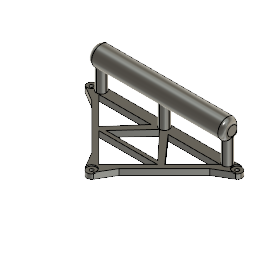
top handle v4 (Autodesk Fusion 360 design; units mm, degrees)
Autodesk Fusion 360 part; units mm, degrees
note: some values were not read from the file. Chosen so that the rebuilt part matches the saved one: which face or edge a step refers to; which pieces of a blend or face edit are solid. Set by a fixed rule: which sketch regions a step uses.
sketch "Sketch1" plane through (0, 0, 0) normal (0, 0, 1) x (1, 0, 0)
  circle A0 centre (0, 0) radius 1.5
  line L0 (0, 0) -> (120, 0)
  circle A1 centre (120, 0) radius 1.5
  circle A2 centre (120, 0) radius 4
  circle A3 centre (0, 0) radius 4
  line L1 (0, 4) -> (0, -4)
  line L2 (120, 4) -> (120, -4)
  line L3 (0, 4) -> (0, -4)
  line L4 (0, -4) -> (9, -4)
  line L5 (9, 4) -> (0, 4)
  line L6 (120, 4) -> (120, -4)
  line L7 (120, -4) -> (111, -4)
  line L8 (111, 4) -> (120, 4)
  line L9 (60, 0) -> (60, -60)
  line L10 (60, -60) -> (120, 0)
  line L11 (0, 0) -> (60, -60)
  line L12 (60, -60) -> (60, -54)
  line L13 (114, 0) -> (60, -54)
  line L14 (6, 0) -> (60, -54)
  line L15 (9, 4) -> (111, 4)
  line L16 (9, -4) -> (111, -4)
  line L17 (60, 0) -> (60, 4)
  circle A4 centre (60, -60) radius 1.5
  circle A5 centre (60, -60) radius 4
  line L18 (0, 0) -> (11.3137, -11.3137)
  line L19 (11.3137, -11.3137) -> (-2.0315, -3.4457)
  line L20 (120, 0) -> (108.6863, -11.3137)
  line L21 (108.6863, -11.3137) -> (122.0315, -3.4457)
  line L22 (60, -60) -> (71.3137, -48.6863)
  line L23 (71.3137, -48.6863) -> (63.4457, -62.0315)
  line L24 (60, -60) -> (48.6863, -48.6863)
  line L25 (48.6863, -48.6863) -> (56.5543, -62.0315)
  line L26 (0, 0) -> (60, -60)
  line L27 (30, -30) -> (60, 4)
  line L28 (30, -30) -> (33.0052, -33.0052)
  line L29 (33.0052, -33.0052) -> (60, -4)
  line L30 (60, -60) -> (120, 0)
  line L31 (90, -30) -> (60, 4)
  line L32 (90, -30) -> (86.9948, -33.0052)
  line L33 (60, -4) -> (86.9948, -33.0052)
  line L34 (35.8975, -29.8975) -> (84.1025, -29.8975)
  line L35 (87.1875, -26.8125) -> (32.8125, -26.8125)
  line L36 (0, 4) -> (12, 4)
  line L37 (12, 4) -> (12, -4)
  line L38 (12, -4) -> (0, -4)
  line L39 (0, -4) -> (0, 4)
  line L40 (12, 4) -> (4, 4)
  line L41 (4, 4) -> (4, -4)
  line L42 (4, -4) -> (12, -4)
  line L43 (12, -4) -> (12, 4)
  line L44 (120, 4) -> (108, 4)
  line L45 (108, 4) -> (108, -4)
  line L46 (108, -4) -> (120, -4)
  line L47 (120, -4) -> (120, 4)
  line L48 (108, 4) -> (116, 4)
  line L49 (116, 4) -> (116, -4)
  line L50 (116, -4) -> (108, -4)
  line L51 (108, -4) -> (108, 4)
  line L52 (64, -4) -> (56, -4)
  line L53 (56, -4) -> (56, 4)
  line L54 (56, 4) -> (64, 4)
  line L55 (64, 4) -> (64, -4)
  line L56 (64, -4) -> (56, 4) construction
  line L57 (56, -4) -> (64, 4) construction
  point P0 (60, 0)
  dimension "d1" = 3
  dimension "d2" = 120
  dimension "d3" = 3
  dimension "d4" = 8
  dimension "d5" = 8
  dimension "d6" = 9
  dimension "d8" = 9
  dimension "d10" = 60
  dimension "d11" = 6
  dimension "d13" = 3
  dimension "d14" = 8
  dimension "d15" = 16
  dimension "d16" = 16
  dimension "d17" = 16
  dimension "d18" = 16
  dimension "d19" = 4.25
  dimension "d20" = 4.25
  dimension "d25" = 12
  dimension "d26" = 8
  dimension "d27" = 8
  dimension "d28" = 12
  dimension "d29" = 8
  dimension "d39" = 8
  constraint coincident A0.centre L0.start
  constraint horizontal L0
  constraint coincident L0.end A1.centre
  constraint concentric A0 A3
  constraint coincident A3 L1.start
  constraint coincident A3 L1.end
  constraint perpendicular L0 L1
  constraint coincident A2 L2.start
  constraint coincident A2 L2.end
  constraint perpendicular L0 L2
  constraint perpendicular L3 L4
  constraint parallel L4 L5
  constraint parallel L1 L3
  constraint perpendicular L6 L7
  constraint parallel L7 L8
  constraint midpoint L0 P0
  constraint perpendicular L0 L9
  constraint parallel L9 L12
  constraint perpendicular L13 L14
  constraint midpoint L15 L17.end
  constraint perpendicular L15 L17
  constraint coincident L9.end L10.start
  constraint parallel L11 L18
  constraint coincident A3 L19.end
  constraint tangent A3 L19
  constraint parallel L10 L20
  constraint coincident A2 L21.end
  constraint tangent A2 L21
  constraint perpendicular L11 L22
  constraint coincident A5 L23.end
  constraint tangent A5 L23
  constraint perpendicular L10 L24
  constraint coincident A5 L25.end
  constraint tangent A5 L25
  constraint midpoint L11 L27.start
  constraint coincident L26 L28.end
  constraint midpoint L16 L29.end
  constraint midpoint L10 L31.start
  constraint coincident L10 L32.end
  constraint coincident L29 L34.start
  constraint coincident L14 L34.start
  constraint coincident L13 L34.end
  constraint coincident L33 L34.end
  constraint coincident L13 L35.start
  constraint coincident L31 L35.start
  constraint coincident L14 L35.end
  constraint coincident L27 L35.end
  constraint horizontal L36
  constraint vertical L37
  constraint horizontal L38
  constraint vertical L39
  constraint horizontal L40
  constraint vertical L41
  constraint horizontal L42
  constraint vertical L43
  constraint coincident L18 L41.end
  constraint horizontal L44
  constraint vertical L45
  constraint horizontal L46
  constraint vertical L47
  constraint coincident L16 L45.end
  constraint horizontal L48
  constraint vertical L49
  constraint horizontal L50
  constraint vertical L51
  constraint coincident L30 L49.end
  constraint perpendicular L52 L53
  constraint parallel L52 L54
  constraint parallel L53 L55
  constraint horizontal L52
  constraint coincident L16 L52.start
  constraint coincident L56 P0
  constraint coincident L57 P0
  constraint coincident P0 L9.start
  measures "d1" diameter of A0
  measures "d2" distance of A0.centre L0.end
  measures "d3" diameter of A1
  measures "d4" diameter of A2
  measures "d5" diameter of A3
  measures "d6" distance of L1.start L5.start
  measures "d8" distance of L2.start L8.start
  measures "d10" distance of P0 L9.end
  measures "d11" distance of L9.end L12.end
  measures "d13" diameter of A4
  measures "d14" diameter of A5
  measures "d15" distance of A0.centre L18.end
  measures "d16" distance of L0.end L20.end
  measures "d17" distance of L9.end L22.end
  measures "d18" distance of L9.end L24.end
  measures "d19" distance of L27.start L28.end
  measures "d20" distance of L31.start L32.end
  measures "d25" distance of L1.start L36.end
  measures "d26" distance of L1.start L1.end
  measures "d27" distance of L36.end L40.end
  measures "d28" distance of L2.start L44.end
  measures "d29" distance of L44.end L48.end
  measures "d39" distance of L53.end L54.end
extrude "Extrude1" add sketch "Sketch1" along normal blind 4 contours A0 L0 A3 L11 L18 L26 | A0 L0 A3 L1 L3 L39 | A0 A3 L1 L3 L39 | A0 A3 L1 L3 L11 L18 L26 L39 | L9 L10 L12 A4 A5 L22 L30 | L9 L11 L12 A4 A5 L24 L26 | L10 L11 A4 A5 L22 L24 L26 L30 | L0 A1 A2 L2 L6 L47 | L0 A1 A2 L10 L20 L30 | A1 A2 L2 L6 L47 | A1 A2 L2 L6 L10 L20 L30 L47 makes body 1 at (63.9801, -59.6017, 2.6667) makes body 2 at (123.995, -0.1994, 1.3333) makes body 3 at (3.995, -0.1994, 1.3333)
extrude "Extrude2" add sketch "Sketch1" along normal blind 5 contours L0 L5 L15 L36 L37 L40 L41 L43 | A3 L11 L18 L26 L41 | A3 L5 L36 L41 | L0 L4 L14 L16 L38 L41 L42 | A3 L4 L11 L18 L26 L38 | L0 L14 L16 L37 L38 L42 L43 | A3 L4 L11 L18 L19 L26 L38 | L4 L11 L14 L16 L18 L26 L27 L38 L42 | L0 L15 L37 L43 L53 | L0 L16 L27 L37 L43 L53 | L0 L15 L27 L53 L54 | L0 L27 L53 | L14 L29 L35 | L11 L14 L26 L27 L28 L29 | L16 L27 L29 L35 L52 | L0 L17 L27 | L0 L9 L16 L27 L52 L53 | L16 L27 L53 | L9 L11 L12 L14 A5 L24 L26 L29 | L9 L29 L34 L35 | L0 L17 L31 | L0 L9 L16 L31 L52 L55 | L0 L15 L31 L54 L55 | L9 L10 L12 L13 A5 L22 L30 L33 | L9 L33 L34 L35 | L16 L31 L33 L35 L52 | L11 A5 L24 L25 L26 | L0 L31 L55 | L0 L15 L45 L51 L55 | L13 L33 L35 | L10 L13 L30 L31 L32 L33 | L16 L31 L55 | L0 L16 L31 L45 L51 L55 | L0 L8 L15 L44 L45 L48 L49 L51 | L10 A5 L22 L23 L30 | L7 L10 L13 L16 L20 L30 L31 L46 L50 | L0 L13 L16 L45 L46 L50 L51 | L0 L7 L13 L16 L46 L49 L50 | A2 L8 L44 L49 | A2 L7 L10 L20 L21 L30 L46 | A2 L10 L20 L30 L49 | A2 L7 L10 L20 L30 L46 bodies 1 2 3
extrude "Extrude3" add sketch "Sketch1" along normal blind 35 contours L0 L5 L15 L36 L37 L40 L41 L43 | L0 L4 L14 L16 L38 L41 L42 | L0 L14 L16 L37 L38 L42 L43 | L0 L8 L15 L44 L45 L48 L49 L51 | L0 L13 L16 L45 L46 L50 L51 | L0 L7 L13 L16 L46 L49 L50 bodies 1
sketch "Sketch5" plane through (116, 0, 0) normal (1, 0, 0) x (0, 1, 0)
  line L0 (-4, 5) -> (0, 5)
  line L1 (0, 5) -> (4, 5)
  line L2 (4, 5) -> (4, 35)
  line L3 (4, 35) -> (-4, 35)
  line L4 (-4, 35) -> (-4, 5)
  line L5 (0, 5) -> (0, 30)
  circle A0 centre (0, 30) radius 8
  dimension "d52" = 25
  dimension "d53" = 16
  constraint coincident L0.end L1.start
  constraint perpendicular L0 L5
  constraint coincident L5.end A0.centre
  measures "d52" distance of L0.end L5.end
  measures "d53" diameter of A0
extrude "Extrude8" add sketch "Sketch5" against normal blind 112 contours L2 L3 L4 A0 | L2 L3 L4 A0 bodies 1
sketch "Sketch6" plane through (0, 0, 5) normal (0, 0, 1) x (-1, 0, 0)
  line L0 (-116, 0) -> (-116, 4)
  line L1 (-116, 4) -> (-110, 4)
  line L2 (-110, 4) -> (-87.1875, 26.8125)
  line L3 (-87.1875, 26.8125) -> (-67.0588, 4)
  line L4 (-67.0588, 4) -> (-108, 4)
  line L5 (-108, 4) -> (-108, -4)
  line L6 (-108, -4) -> (-12, -4)
  line L7 (-12, -4) -> (-12, 4)
  line L8 (-12, 4) -> (-52.9412, 4)
  line L9 (-52.9412, 4) -> (-32.8125, 26.8125)
  line L10 (-32.8125, 26.8125) -> (-10, 4)
  line L11 (-10, 4) -> (-4, 4)
  line L12 (-4, 4) -> (-4, 0)
  arc A0 (2.0315, 3.4457) -> (-4, 0) centre (0, 0) ccw
  line L13 (2.0315, 3.4457) -> (-11.3137, 11.3137)
  line L14 (-11.3137, 11.3137) -> (-48.6863, 48.6863)
  line L15 (-48.6863, 48.6863) -> (-56.5543, 62.0315)
  arc A1 (-63.4457, 62.0315) -> (-56.5543, 62.0315) centre (-60, 60) ccw
  line L16 (-63.4457, 62.0315) -> (-71.3137, 48.6863)
  line L17 (-71.3137, 48.6863) -> (-108.6863, 11.3137)
  line L18 (-108.6863, 11.3137) -> (-122.0315, 3.4457)
  arc A2 (-116, 0) -> (-122.0315, 3.4457) centre (-120, 0) ccw
  line L19 (-60, 54) -> (-35.8975, 29.8975)
  line L20 (-35.8975, 29.8975) -> (-84.1025, 29.8975)
  line L21 (-84.1025, 29.8975) -> (-60, 54)
  line L22 (-38.7687, 26.8125) -> (-60, 4)
  line L23 (-60, 4) -> (-81.2313, 26.8125)
  line L24 (-81.2313, 26.8125) -> (-38.7687, 26.8125)
  line L25 (-60, 4) -> (-60, -4)
  line L26 (-64, -4) -> (-56, -4)
  line L27 (-56, -4) -> (-56, 4)
  line L28 (-56, 4) -> (-64, 4)
  line L29 (-64, 4) -> (-64, -4)
  line L30 (-64, -4) -> (-56, 4) construction
  line L31 (-56, -4) -> (-64, 4) construction
  point P0 (-60, 0)
  dimension "d56" = 8
  dimension "d57" = 8
  constraint coincident L22.end L23.start
  constraint midpoint L6 L25.end
  constraint perpendicular L26 L27
  constraint parallel L26 L28
  constraint parallel L27 L29
  constraint horizontal L26
  constraint coincident L30 P0
  constraint coincident L31 P0
  constraint midpoint L25 P0
  measures "d56" distance of L26.end L27.end
  measures "d57" distance of L27.end L28.end
extrude "Extrude9" add sketch "Sketch6" along normal blind 25 contours L6 L25 L26 L28 L29 | L6 L25 L26 L27 L28 bodies 1
fillet "Fillet4" radius 3.9999 14 edges at (4, -4, 14.0359) (4, 4, 14.0359) (4, 0, 38) (12, -4, 14.0359) (12, 4, 14.0359) (56, -4, 14.0359) (64, -4, 14.0359) (64, 4, 14.0359) (108, -4, 14.0359) (116, -4, 14.0359) (116, 0, 38) (116, 4, 14.0359) (108, 4, 14.0359) (56, 4, 14.0359) on bodies 1
sketch "Sketch7" plane through (0, 0, 5) normal (0, 0, 1) x (-1, 0, 0)
  line L0 (-110, 4) -> (-87.1875, 26.8125)
  line L1 (-87.1875, 26.8125) -> (-67.0588, 4)
  line L2 (-67.0588, 4) -> (-110, 4)
  line L3 (-10, 4) -> (-52.9412, 4)
  line L4 (-52.9412, 4) -> (-32.8125, 26.8125)
  line L5 (-32.8125, 26.8125) -> (-10, 4)
  arc A0 (-108, 0.0001) -> (-111.9999, 4) centre (-111.9999, 0.0001) ccw
  line L6 (-108, 0.0001) -> (-108, -0.0001)
  arc A1 (-111.9999, -4) -> (-108, -0.0001) centre (-111.9999, -0.0001) ccw
  line L7 (-111.9999, -4) -> (-60.0001, -4)
  arc A2 (-64, -0.0001) -> (-60.0001, -4) centre (-60.0001, -0.0001) ccw
  line L8 (-64, -0.0001) -> (-64, 0.0001)
  arc A3 (-60.0001, 4) -> (-64, 0.0001) centre (-60.0001, 0.0001) ccw
  line L9 (-60.0001, 4) -> (-60, 4)
  line L10 (-60, 4) -> (-81.2313, 26.8125)
  line L11 (-81.2313, 26.8125) -> (-38.7687, 26.8125)
  line L12 (-38.7687, 26.8125) -> (-60, 4)
  line L13 (-60, 4) -> (-59.9999, 4)
  arc A4 (-56, 0.0001) -> (-59.9999, 4) centre (-59.9999, 0.0001) ccw
  line L14 (-56, 0.0001) -> (-56, -0.0001)
  arc A5 (-59.9999, -4) -> (-56, -0.0001) centre (-59.9999, -0.0001) ccw
  line L15 (-59.9999, -4) -> (-8.0001, -4)
  arc A6 (-12, -0.0001) -> (-8.0001, -4) centre (-8.0001, -0.0001) ccw
  line L16 (-12, -0.0001) -> (-12, 0.0001)
  arc A7 (-8.0001, 4) -> (-12, 0.0001) centre (-8.0001, 0.0001) ccw
  line L17 (-8.0001, 4) -> (-7.9999, 4)
  arc A8 (-4, 0.0001) -> (-7.9999, 4) centre (-7.9999, 0.0001) ccw
  line L18 (-4, 0.0001) -> (-4, 0)
  arc A9 (2.0315, 3.4457) -> (-4, 0) centre (0, 0) ccw
  line L19 (2.0315, 3.4457) -> (-11.3137, 11.3137)
  line L20 (-11.3137, 11.3137) -> (-48.6863, 48.6863)
  line L21 (-48.6863, 48.6863) -> (-56.5543, 62.0315)
  arc A10 (-63.4457, 62.0315) -> (-56.5543, 62.0315) centre (-60, 60) ccw
  line L22 (-63.4457, 62.0315) -> (-71.3137, 48.6863)
  line L23 (-71.3137, 48.6863) -> (-108.6863, 11.3137)
  line L24 (-108.6863, 11.3137) -> (-122.0315, 3.4457)
  arc A11 (-116, 0) -> (-122.0315, 3.4457) centre (-120, 0) ccw
  line L25 (-116, 0) -> (-116, 0.0001)
  arc A12 (-112.0001, 4) -> (-116, 0.0001) centre (-112.0001, 0.0001) ccw
  line L26 (-112.0001, 4) -> (-111.9999, 4)
  line L27 (-60, 54) -> (-35.8975, 29.8975)
  line L28 (-35.8975, 29.8975) -> (-84.1025, 29.8975)
  line L29 (-84.1025, 29.8975) -> (-60, 54)
  line L30 (0, -4) -> (-116.6971, -4)
  line L31 (-116.6971, -4) -> (-116.6971, -14.5936)
  line L32 (-116.6971, -14.5936) -> (0, -14.5936)
  line L33 (0, -14.5936) -> (0, -4)
  point P0 (0, -4)
  constraint horizontal L30
  constraint vertical L31
  constraint horizontal L32
  constraint vertical L33
  constraint coincident P0 L30.start
extrude "Extrude10" cut sketch "Sketch7" along normal blind 50 contours L7 L15 L30 L31 L32 L33 bodies 1
sketch "Sketch2" plane through (116, 0, 0) normal (1, 0, 0) x (0, 1, 0)
  line L0 (4, 5) -> (4, 30)
  line L1 (4, 30) -> (-4, 30)
  line L2 (-4, 30) -> (-4, 5)
  line L3 (0, 30) -> (0, 26)
  circle A0 centre (0, 26) radius 6
  line L4 (-4, 5) -> (0, 5)
  line L5 (0, 5) -> (4, 5)
  dimension "d32" = 4
  dimension "d33" = 12
  constraint midpoint L1 L3.start
  constraint perpendicular L1 L3
  constraint coincident L3.end A0.centre
  measures "d32" distance of L3.start L3.end
  measures "d33" diameter of A0
extrude "Extrude4" [suppressed]
fillet "Fillet1" [suppressed]
sketch "Sketch3" plane through (0, 0, 0) normal (0, 0, 1) x (1, 0, 0)
  line L0 (0, 4) -> (120, 4)
  line L1 (120, 4) -> (120, 12)
  line L2 (120, 12) -> (0, 12)
  line L3 (0, 12) -> (0, 4)
  point P0 (0, 4)
  dimension "d37" = 120
  dimension "d38" = 8
  constraint horizontal L0
  constraint vertical L1
  constraint horizontal L2
  constraint vertical L3
  measures "d37" distance of P0 L0.end
  measures "d38" distance of P0 L2.end
extrude "Extrude5" [suppressed]
fillet "Fillet2" [suppressed]
extrude "Extrude6" [suppressed]
extrude "Extrude7" [suppressed]
fillet "Fillet3" [suppressed]
